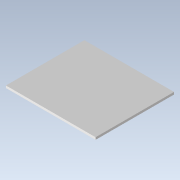
# Autodesk Inventor part: platina_1
Saved by Autodesk Inventor 2021 (Build 250183000, 183)
## iProperties
Created: 2021-04-25
Part Number: platina_1
Material: Genérico
Document SubType Name: Modeling
Designer: j2seb
Density: 1 g/cm^3
Appearance: Valor por defecto
Author: j2seb
Autodesk Inventor part; units mm, degrees
ref_plane "YZ Plane" through (0, 0, 0) normal (1, 0, 0) x (0, 1, 0)
ref_plane "XZ Plane" through (0, 0, 0) normal (0, 1, 0) x (-1, 0, 0)
ref_plane "XY Plane" through (0, 0, 0) normal (0, 0, 1) x (1, 0, 0)
sketch "Boceto1" plane through (0, 0, 0) normal (0, 1, 0) x (-1, 0, 0)
  line L0 (0, 0) -> (0, -40)
  line L1 (0, -40) -> (60, -40)
  line L2 (60, 0) -> (0, 0)
  line L3 (60, -40) -> (60, 0)
  dimension "d1" = 60
  dimension "d3" = 40
  constraints: 8 end point, 2 vertical, 1 horizontal, 1 parallel, 1 vertical alignment
  measures "d1" distance of L0.end L1.end
  measures "d3" distance of L0.start L0.end
extrude "Extrusión1" add sketch "Boceto1" along normal blind 1
sketch "Boceto2" plane through (0, 0, 0) normal (0, -1, 0) x (1, 0, 0)
  line L0 (0, 0) -> (0, -40) projected
  circle A0 centre (9, -20) radius 22
  point P0 (0, -20)
  dimension "d7" = 44
  dimension "d8" = 9
  constraints: 1 centre point, 1 horizontal alignment, 1 midpoint
  measures "d7" diameter of A0
  measures "d8" distance from line of A0.centre L0
extrude "Extrusión2" cut sketch "Boceto2" against normal through all
